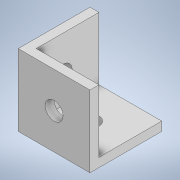
# Autodesk Inventor part: MountingBracket
Saved by Autodesk Inventor 2020 (Build 240168000, 168)
## iProperties
Created: 2022-01-23
Part Number: MountingBracket
Material: Generic
Document SubType Name: Modeling
Designer: danie
Density: 1 g/cm^3
Appearance: Default
Author: danie
Autodesk Inventor part; units mm, degrees
ref_plane "YZ Plane" through (0, 0, 0) normal (1, 0, 0) x (0, 1, 0)
ref_plane "XZ Plane" through (0, 0, 0) normal (0, 1, 0) x (-1, 0, 0)
ref_plane "XY Plane" through (0, 0, 0) normal (0, 0, 1) x (1, 0, 0)
sketch "Sketch1" plane through (0, 0, 0) normal (0, 1, 0) x (-1, 0, 0)
  line L0 (0, 0) -> (-25.4, 0)
  line L1 (-25.4, 0) -> (-25.4, -25.4)
  line L2 (-25.4, -25.4) -> (0, -25.4)
  line L3 (0, -25.4) -> (0, 0)
  line L4 (0, 0) -> (-25.4, -25.4) construction
  line L5 (0, -25.4) -> (-25.4, 0) construction
  circle A0 centre (-12.7, -12.7) radius 3.175
  dimension "d0" = 25.4
  dimension "d1" = 25.4
  dimension "d2" = 6.35
  constraints: 12 end point, 2 parallel, 1 centre point, 1 horizontal, 1 midpoint, 1 perpendicular
  measures "d0" distance of L2.end L1.end
  measures "d1" distance of L1.end L0.end
  measures "d2" diameter of A0
extrude "Extrusion1" add sketch "Sketch1" along normal blind 3.175
sketch "Sketch2" plane through (0, 0, 0) normal (0, 0, 1) x (1, 0, 0)
  line L0 (0, 0) -> (0, 3.175) projected
  line L1 (0, 0) -> (25.4, 0)
  line L2 (25.4, 0) -> (25.4, 25.4)
  line L3 (25.4, 25.4) -> (0, 25.4)
  line L4 (0, 25.4) -> (0, 0)
  line L5 (25.4, 0) -> (25.4, 3.175) construction
  line L6 (0, 25.4) -> (25.4, 0) construction
  line L7 (25.4, 25.4) -> (0, 0) construction
  circle A0 centre (12.7, 12.7) radius 3.175
  dimension "d5" = 25.4
  dimension "d6" = 25.4
  dimension "d7" = 6.35
  constraints: 12 end point, 2 parallel, 1 centre point, 1 horizontal, 1 midpoint, 1 perpendicular
  measures "d5" distance of L3.end L2.end
  measures "d6" distance of L2.end L1.end
  measures "d7" diameter of A0
extrude "Extrusion2" add sketch "Sketch2" against normal blind 3.175
sketch "Sketch3" plane through (0, 0, -25.4) normal (-1, 0, 0) x (0, 0, 1)
  line L0 (0, 0) -> (25.4, 0) projected
  line L1 (25.4, 0) -> (25.4, 25.4) projected
  line L2 (0, 0) -> (25.4, 0)
  line L3 (25.4, 0) -> (25.4, 25.4)
  line L4 (25.4, 25.4) -> (0, 25.4)
  line L5 (0, 25.4) -> (0, 0)
  line L6 (0, 25.4) -> (25.4, 0) construction
  line L7 (25.4, 25.4) -> (0, 0) construction
  circle A0 centre (12.7, 12.7) radius 3.175
  dimension "d10" = 25.4
  dimension "d11" = 6.35
  constraints: 12 end point, 2 parallel, 2 perpendicular, 1 centre point, 1 horizontal, 1 midpoint
  measures "d10" distance of L4.end L1.end
  measures "d11" diameter of A0
extrude "Extrusion3" add sketch "Sketch3" against normal blind 3.175
body "Solid1"
